Autodesk Fusion 360 part; units mm, degrees
(part 5 of 6)
sketch "Sketch13" plane through (0, 0, 0) normal (0, -1, 0) x (1, 0, 0)
  line L0 (140.1031, 86.5919) -> (126.1031, 86.5919)
  line L1 (126.1031, 86.5919) -> (126.1031, 100.5919)
  line L2 (126.1031, 100.5919) -> (140.1031, 100.5919)
  line L3 (140.1031, 100.5919) -> (140.1031, 86.5919)
  line L4 (30.8531, 93.7533) -> (30.8531, 107.7533)
  line L5 (30.8531, 107.7533) -> (44.8531, 107.7533)
  line L6 (44.8531, 107.7533) -> (44.8531, 93.7533)
  line L7 (44.8531, 93.7533) -> (30.8531, 93.7533)
  line L8 (126.1031, 67.5419) -> (126.1031, 81.5419)
  line L9 (126.1031, 81.5419) -> (140.1031, 81.5419)
  line L10 (140.1031, 81.5419) -> (140.1031, 67.5419)
  line L11 (140.1031, 67.5419) -> (126.1031, 67.5419)
  line L12 (49.9031, 98.5158) -> (49.9031, 112.5158)
  line L13 (49.9031, 112.5158) -> (63.9031, 112.5158)
  line L14 (63.9031, 112.5158) -> (63.9031, 98.5158)
  line L15 (63.9031, 98.5158) -> (49.9031, 98.5158)
  line L16 (107.0531, 96.1169) -> (107.0531, 110.1169)
  line L17 (107.0531, 110.1169) -> (121.0531, 110.1169)
  line L18 (121.0531, 110.1169) -> (121.0531, 96.1169)
  line L19 (121.0531, 96.1169) -> (107.0531, 96.1169)
  line L20 (11.8031, 93.7533) -> (11.8031, 107.7533)
  line L21 (11.8031, 107.7533) -> (25.8031, 107.7533)
  line L22 (25.8031, 107.7533) -> (25.8031, 93.7533)
  line L23 (25.8031, 93.7533) -> (11.8031, 93.7533)
  line L24 (49.9031, 41.3658) -> (49.9031, 55.3658)
  line L25 (49.9031, 55.3658) -> (63.9031, 55.3658)
  line L26 (63.9031, 55.3658) -> (63.9031, 41.3658)
  line L27 (63.9031, 41.3658) -> (49.9031, 41.3658)
  line L28 (30.8531, 74.7033) -> (30.8531, 88.7033)
  line L29 (30.8531, 88.7033) -> (44.8531, 88.7033)
  line L30 (44.8531, 88.7033) -> (44.8531, 74.7033)
  line L31 (44.8531, 74.7033) -> (30.8531, 74.7033)
  line L32 (30.8531, 55.6533) -> (30.8531, 69.6533)
  line L33 (30.8531, 69.6533) -> (44.8531, 69.6533)
  line L34 (44.8531, 69.6533) -> (44.8531, 55.6533)
  line L35 (44.8531, 55.6533) -> (30.8531, 55.6533)
  line L36 (11.8031, 17.5533) -> (11.8031, 31.5533)
  line L37 (11.8031, 31.5533) -> (25.8031, 31.5533)
  line L38 (25.8031, 31.5533) -> (25.8031, 17.5533)
  line L39 (25.8031, 17.5533) -> (11.8031, 17.5533)
  line L40 (116.8975, 10.2287) -> (104.7731, 17.2287)
  line L41 (104.7731, 17.2287) -> (106.7731, 20.6928)
  line L42 (106.7731, 20.6928) -> (104.9761, 21.7303)
  line L43 (104.9761, 21.7303) -> (103.3761, 18.959)
  line L44 (103.3761, 18.959) -> (98.3098, 21.884)
  line L45 (98.3098, 21.884) -> (104.5098, 32.6227)
  line L46 (104.5098, 32.6227) -> (109.5761, 29.6977)
  line L47 (109.5761, 29.6977) -> (107.9761, 26.9264)
  line L48 (107.9761, 26.9264) -> (109.7731, 25.8889)
  line L49 (109.7731, 25.8889) -> (111.7731, 29.353)
  line L50 (111.7731, 29.353) -> (123.8975, 22.353)
  line L51 (123.8975, 22.353) -> (121.8975, 18.8889)
  line L52 (121.8975, 18.8889) -> (123.6945, 17.8514)
  line L53 (123.6945, 17.8514) -> (125.2945, 20.6227)
  line L54 (125.2945, 20.6227) -> (130.3607, 17.6977)
  line L55 (130.3607, 17.6977) -> (124.1607, 6.959)
  line L56 (124.1607, 6.959) -> (119.0945, 9.884)
  line L57 (119.0945, 9.884) -> (120.6945, 12.6553)
  line L58 (120.6945, 12.6553) -> (118.8975, 13.6928)
  line L59 (118.8975, 13.6928) -> (116.8975, 10.2287)
  line L60 (30.8531, 36.6033) -> (30.8531, 50.6033)
  line L61 (30.8531, 50.6033) -> (44.8531, 50.6033)
  line L62 (44.8531, 50.6033) -> (44.8531, 36.6033)
  line L63 (44.8531, 36.6033) -> (30.8531, 36.6033)
  line L64 (11.8031, 36.6033) -> (11.8031, 50.6033)
  line L65 (11.8031, 50.6033) -> (25.8031, 50.6033)
  line L66 (25.8031, 50.6033) -> (25.8031, 36.6033)
  line L67 (25.8031, 36.6033) -> (11.8031, 36.6033)
  line L68 (11.8031, 55.6533) -> (11.8031, 69.6533)
  line L69 (11.8031, 69.6533) -> (25.8031, 69.6533)
  line L70 (25.8031, 69.6533) -> (25.8031, 55.6533)
  line L71 (25.8031, 55.6533) -> (11.8031, 55.6533)
  line L72 (11.8031, 74.7033) -> (11.8031, 88.7033)
  line L73 (11.8031, 88.7033) -> (25.8031, 88.7033)
  line L74 (25.8031, 88.7033) -> (25.8031, 74.7033)
  line L75 (25.8031, 74.7033) -> (11.8031, 74.7033)
  line L76 (134.7127, 21.9762) -> (122.5884, 28.9762)
  line L77 (122.5884, 28.9762) -> (129.5884, 41.1005)
  line L78 (129.5884, 41.1005) -> (141.7127, 34.1005)
  line L79 (141.7127, 34.1005) -> (134.7127, 21.9762)
  line L80 (141.6977, -4.0941) -> (129.5734, 2.9059)
  line L81 (129.5734, 2.9059) -> (136.5734, 15.0302)
  line L82 (136.5734, 15.0302) -> (148.6977, 8.0302)
  line L83 (148.6977, 8.0302) -> (141.6977, -4.0941)
  line L84 (30.8531, 17.5533) -> (30.8531, 31.5533)
  line L85 (30.8531, 31.5533) -> (44.8531, 31.5533)
  line L86 (44.8531, 31.5533) -> (44.8531, 17.5533)
  line L87 (44.8531, 17.5533) -> (30.8531, 17.5533)
  line L88 (49.9031, 22.3158) -> (49.9031, 36.3158)
  line L89 (49.9031, 36.3158) -> (63.9031, 36.3158)
  line L90 (63.9031, 36.3158) -> (63.9031, 22.3158)
  line L91 (63.9031, 22.3158) -> (49.9031, 22.3158)
  line L92 (68.9531, 100.8794) -> (68.9531, 114.8794)
  line L93 (68.9531, 114.8794) -> (82.9531, 114.8794)
  line L94 (82.9531, 114.8794) -> (82.9531, 100.8794)
  line L95 (82.9531, 100.8794) -> (68.9531, 100.8794)
  line L96 (68.9531, 81.8294) -> (68.9531, 95.8294)
  line L97 (68.9531, 95.8294) -> (82.9531, 95.8294)
  line L98 (82.9531, 95.8294) -> (82.9531, 81.8294)
  line L99 (82.9531, 81.8294) -> (68.9531, 81.8294)
  line L100 (68.9531, 62.7794) -> (68.9531, 76.7794)
  line L101 (68.9531, 76.7794) -> (82.9531, 76.7794)
  line L102 (82.9531, 76.7794) -> (82.9531, 62.7794)
  line L103 (82.9531, 62.7794) -> (68.9531, 62.7794)
  line L104 (68.9531, 43.7294) -> (68.9531, 57.7294)
  line L105 (68.9531, 57.7294) -> (82.9531, 57.7294)
  line L106 (82.9531, 57.7294) -> (82.9531, 43.7294)
  line L107 (82.9531, 43.7294) -> (68.9531, 43.7294)
  line L108 (76.5731, 22.3158) -> (76.5731, 36.3158)
  line L109 (76.5731, 36.3158) -> (90.5731, 36.3158)
  line L110 (90.5731, 36.3158) -> (90.5731, 22.3158)
  line L111 (90.5731, 22.3158) -> (76.5731, 22.3158)
  line L112 (49.9031, 60.4158) -> (49.9031, 74.4158)
  line L113 (49.9031, 74.4158) -> (63.9031, 74.4158)
  line L114 (63.9031, 74.4158) -> (63.9031, 60.4158)
  line L115 (63.9031, 60.4158) -> (49.9031, 60.4158)
  line L116 (49.9031, 79.4658) -> (49.9031, 93.4658)
  line L117 (49.9031, 93.4658) -> (63.9031, 93.4658)
  line L118 (63.9031, 93.4658) -> (63.9031, 79.4658)
  line L119 (63.9031, 79.4658) -> (49.9031, 79.4658)
  line L120 (126.1031, 48.4919) -> (126.1031, 62.4919)
  line L121 (126.1031, 62.4919) -> (140.1031, 62.4919)
  line L122 (140.1031, 62.4919) -> (140.1031, 48.4919)
  line L123 (140.1031, 48.4919) -> (126.1031, 48.4919)
  line L124 (88.0031, 60.4158) -> (88.0031, 74.4158)
  line L125 (88.0031, 74.4158) -> (102.0031, 74.4158)
  line L126 (102.0031, 74.4158) -> (102.0031, 60.4158)
  line L127 (102.0031, 60.4158) -> (88.0031, 60.4158)
  line L128 (107.0531, 91.0669) -> (121.0531, 91.0669)
  line L129 (121.0531, 91.0669) -> (121.0531, 77.0669)
  line L130 (121.0531, 77.0669) -> (107.0531, 77.0669)
  line L131 (107.0531, 77.0669) -> (107.0531, 91.0669)
  line L132 (88.0031, 79.4658) -> (88.0031, 93.4658)
  line L133 (88.0031, 93.4658) -> (102.0031, 93.4658)
  line L134 (102.0031, 93.4658) -> (102.0031, 79.4658)
  line L135 (102.0031, 79.4658) -> (88.0031, 79.4658)
  line L136 (107.0531, 58.0169) -> (107.0531, 72.0169)
  line L137 (107.0531, 72.0169) -> (121.0531, 72.0169)
  line L138 (121.0531, 72.0169) -> (121.0531, 58.0169)
  line L139 (121.0531, 58.0169) -> (107.0531, 58.0169)
  line L140 (107.0531, 38.9669) -> (107.0531, 52.9669)
  line L141 (107.0531, 52.9669) -> (121.0531, 52.9669)
  line L142 (121.0531, 52.9669) -> (121.0531, 38.9669)
  line L143 (121.0531, 38.9669) -> (107.0531, 38.9669)
  line L144 (88.0031, 41.3658) -> (88.0031, 55.3658)
  line L145 (88.0031, 55.3658) -> (102.0031, 55.3658)
  line L146 (102.0031, 55.3658) -> (102.0031, 41.3658)
  line L147 (102.0031, 41.3658) -> (88.0031, 41.3658)
  circle A0 centre (71.0494, 18.8031) radius 1.1
  line L148 (102.0031, 112.5158) -> (102.0031, 98.5158)
  line L149 (102.0031, 98.5158) -> (88.0031, 98.5158)
  line L150 (88.0031, 98.5158) -> (88.0031, 112.5158)
  line L151 (88.0031, 112.5158) -> (102.0031, 112.5158)
  circle A1 centre (18.8031, 34.0783) radius 1.1
  circle A2 centre (28.3281, 91.2283) radius 1.1
  circle A3 centre (95.25, 34.2547) radius 1.1
  circle A4 centre (115.7464, 33.7256) radius 1.1
  circle A5 centre (146.7556, 76.7997) radius 1.1
  circle A6 centre (157.6917, 44.4147) radius 1.1
  circle A7 centre (146.7556, 37.8883) radius 1.1
  line L152 (151.2227, 12.4159) -> (139.0984, 19.4159)
  line L153 (139.0984, 19.4159) -> (146.0984, 31.5402)
  line L154 (146.0984, 31.5402) -> (158.2227, 24.5402)
  line L155 (158.2227, 24.5402) -> (151.2227, 12.4159)
  circle A8 centre (123.5781, 102.5878) radius 1.1
  circle A9 centre (66.4281, 78.105) radius 1.1
  circle A10 centre (130.9158, 10.2658) radius 1.1
  arc A11 (142.7339, 99.2011) -> (138.7122, 103.2228) centre (138.7122, 99.2011) ccw
  line L156 (138.7122, 103.2228) -> (132.5162, 103.2228)
  arc A12 (131.5417, 103.3426) -> (132.5162, 103.2228) centre (132.5162, 107.2444) ccw
  line L157 (131.5417, 103.3426) -> (126.6957, 104.553)
  arc A13 (123.6486, 108.4548) -> (126.6957, 104.553) centre (127.6703, 108.4548) ccw
  line L158 (123.6486, 108.4548) -> (123.6486, 112.6772)
  line L159 (123.6486, 112.6772) -> (84.9842, 117.4397)
  line L160 (84.9842, 117.4397) -> (66.9572, 117.4397)
  line L161 (66.9572, 117.4397) -> (9.2428, 110.3136)
  line L162 (9.2428, 110.3136) -> (9.2428, 14.9931)
  line L163 (9.2428, 14.9931) -> (103.8578, 14.9931)
  line L164 (103.8578, 14.9931) -> (142.6281, -7.5847)
  line L165 (142.6281, -7.5847) -> (161.7839, 25.5411)
  arc A14 (150.7772, 34.2581) -> (152.8134, 30.7285) centre (154.8544, 34.2581) ccw
  line L166 (150.7772, 34.2581) -> (150.7772, 36.2632)
  arc A15 (154.8573, 40.3375) -> (150.7772, 36.2632) centre (154.8544, 36.2603) ccw
  line L167 (154.8573, 40.3375) -> (157.6917, 40.3375)
  arc A16 (157.6917, 40.3375) -> (157.6917, 48.4919) centre (157.6917, 44.4147) ccw
  line L168 (157.6917, 48.4919) -> (146.8111, 48.4919)
  arc A17 (142.7339, 52.5692) -> (146.8111, 48.4919) centre (146.8111, 52.5692) ccw
  line L169 (142.7339, 52.5692) -> (142.7339, 68.7564)
  arc A18 (146.7556, 72.7781) -> (142.7339, 68.7564) centre (146.7556, 68.7564) ccw
  arc A19 (146.7556, 72.7781) -> (146.7556, 80.8214) centre (146.7556, 76.7997) ccw
  arc A20 (142.7339, 84.843) -> (146.7556, 80.8214) centre (146.7556, 84.843) ccw
  line L170 (142.7339, 84.843) -> (142.7339, 99.2011)
  circle A21 centre (239.7, 32.1911) radius 17.4978
  circle A22 centre (239.7, 32.1911) radius 22.2956
  circle A23 centre (243.8628, 51.6644) radius 1.5169
  circle A24 centre (254.8342, 19.2794) radius 1.5169
  circle A25 centre (243.8628, 12.7531) radius 1.5169
  line L171 (239.7, 32.1911) -> (239.7, -10)
  line L172 (239.7, 32.1911) -> (243.8628, 12.7531)
  line L173 (239.7, 32.1911) -> (254.8342, 19.2794)
  line L174 (239.7, 32.1911) -> (243.8628, 51.6644)
  circle A26 centre (141.6031, 57.8929) radius 24.599
  circle A27 centre (141.6031, 57.8929) radius 17.5
  circle A28 centre (146.7556, 76.7997) radius 1.1
  circle A29 centre (157.6917, 44.4147) radius 1.1
  circle A30 centre (146.7556, 37.8883) radius 1.1
  line L175 (141.6031, 57.8929) -> (141.6031, 33.2939)
  line L176 (146.7556, 76.7997) -> (141.6031, 57.8929)
  line L177 (146.7556, 37.8883) -> (141.6031, 57.8929)
  line L178 (141.6031, 57.8929) -> (124.1031, 57.8929)
  line L179 (141.6031, 57.8929) -> (161.7839, 57.8929)
  line L180 (161.7839, 103.1522) -> (161.7839, 25.5411)
  line L181 (161.7839, 71.9587) -> (161.7839, 43.8272)
  line L182 (161.7839, 43.8272) -> (161.7839, 25.5411)
  line L183 (123.0531, 54.9669) -> (123.0531, 36.9669)
  line L184 (123.0531, 74.0169) -> (123.0531, 56.0169)
  line L185 (124.1031, 57.8929) -> (124.1031, 75.1805)
  line L186 (147.8246, 34.0937) -> (132.8531, 42.7375)
  line L187 (128.8563, 43.8326) -> (144.4448, 34.8326)
  line L188 (105.0531, 74.0169) -> (123.0531, 74.0169)
  line L189 (105.0531, 54.9669) -> (123.0531, 54.9669)
  line L190 (123.0531, 56.0169) -> (105.0531, 56.0169)
  line L191 (142.1031, 84.5919) -> (124.1031, 84.5919)
  line L192 (130.661, 82.4919) -> (167, 82.4919)
  point P0 (257.1978, 32.1911)
  point P1 (261.9956, 32.1911)
  point P2 (245.3797, 51.6644)
  point P3 (256.3511, 19.2794)
  point P4 (245.3797, 12.7531)
  point P5 (124.1031, 57.8929)
  dimension "d564" = 34.9956
  dimension "d565" = 44.5911
  dimension "d566" = 12.088
  dimension "d567" = 49.531
  dimension "d568" = 167.934
  dimension "d570" = 35
  dimension "d582" = 1.05
  dimension "d583" = 1.05
  dimension "d584" = 1.05
  dimension "d585" = 2.1
  constraint coincident A21.centre A22.centre
  constraint vertical L171
  constraint coincident A25.centre L172.end
  constraint coincident A24.centre L173.end
  constraint coincident A23.centre L174.end
  constraint concentric A26 A27
  constraint coincident A26.centre A27.centre
  constraint coincident A26 L175.end
  constraint parallel L169 L175
  constraint coincident A5.centre A19.centre
  constraint coincident A7.centre A30.centre
  constraint perpendicular L120 L178
  constraint perpendicular L175 L179
  constraint coincident L179.end L180
  constraint coincident L180 L181.start
  constraint coincident A26 L181.start
  constraint coincident L180 L181.end
  constraint coincident A26 L181.end
  constraint coincident A27 P5
  constraint coincident L178 P5
  constraint coincident P5 L178.end
  constraint coincident A26 L185.end
  constraint tangent A27 L185
  constraint perpendicular L178 L185
  constraint parallel L186 L187
  constraint coincident A27 L186.end
  constraint coincident A26 L186.start
  constraint tangent A27 L186
  constraint perpendicular L10 L192
  constraint tangent A26 L192
  measures "d564" diameter of A21
  measures "d565" diameter of A22
  measures "d566" angle of L171 L172
  measures "d567" angle of L171 L173
  measures "d568" angle of L171 L174
  measures "d570" diameter of A27
  measures "d582" distance of L189 L190
  measures "d583" distance of L184 L185
  measures "d584" distance of L186 L187
  measures "d585" distance of L191 L192
extrude "Extrude10" add sketch "Sketch13" against normal blind 1.2 from surface at 9.7 separate body contours L8 L11 A26 A27 L185 | L8 L9 L10 L11 A26 A27 | L9 L10 A19 A20 A26 A27 | A19 A20 A26 A27 L179 L180 L181 | A16 L168 A26 A27 L179 L180 L181 | A27 L175 L186 | L166 A15 L167 A16 L168 A26 A27 L175 L186 | L166 A15 L167 A16 A26 makes body 47
fillet "Fillet1" radius 0.5 2 edges at (124.1031, -9.1, 57.8929) (132.8531, -9.1, 42.7375) on bodies 47
sketch "Sketch14" plane through (0, 0, 0) normal (0, -1, 0) x (1, 0, 0)
  line L0 (140.1031, 86.5919) -> (126.1031, 86.5919)
  line L1 (126.1031, 86.5919) -> (126.1031, 100.5919)
  line L2 (126.1031, 100.5919) -> (140.1031, 100.5919)
  line L3 (140.1031, 100.5919) -> (140.1031, 86.5919)
  line L4 (30.8531, 93.7533) -> (30.8531, 107.7533)
  line L5 (30.8531, 107.7533) -> (44.8531, 107.7533)
  line L6 (44.8531, 107.7533) -> (44.8531, 93.7533)
  line L7 (44.8531, 93.7533) -> (30.8531, 93.7533)
  line L8 (126.1031, 67.5419) -> (126.1031, 81.5419)
  line L9 (126.1031, 81.5419) -> (140.1031, 81.5419)
  line L10 (140.1031, 81.5419) -> (140.1031, 67.5419)
  line L11 (140.1031, 67.5419) -> (126.1031, 67.5419)
  line L12 (49.9031, 98.5158) -> (49.9031, 112.5158)
  line L13 (49.9031, 112.5158) -> (63.9031, 112.5158)
  line L14 (63.9031, 112.5158) -> (63.9031, 98.5158)
  line L15 (63.9031, 98.5158) -> (49.9031, 98.5158)
  line L16 (107.0531, 96.1169) -> (107.0531, 110.1169)
  line L17 (107.0531, 110.1169) -> (121.0531, 110.1169)
  line L18 (121.0531, 110.1169) -> (121.0531, 96.1169)
  line L19 (121.0531, 96.1169) -> (107.0531, 96.1169)
  line L20 (11.8031, 93.7533) -> (11.8031, 107.7533)
  line L21 (11.8031, 107.7533) -> (25.8031, 107.7533)
  line L22 (25.8031, 107.7533) -> (25.8031, 93.7533)
  line L23 (25.8031, 93.7533) -> (11.8031, 93.7533)
  line L24 (49.9031, 41.3658) -> (49.9031, 55.3658)
  line L25 (49.9031, 55.3658) -> (63.9031, 55.3658)
  line L26 (63.9031, 55.3658) -> (63.9031, 41.3658)
  line L27 (63.9031, 41.3658) -> (49.9031, 41.3658)
  line L28 (30.8531, 74.7033) -> (30.8531, 88.7033)
  line L29 (30.8531, 88.7033) -> (44.8531, 88.7033)
  line L30 (44.8531, 88.7033) -> (44.8531, 74.7033)
  line L31 (44.8531, 74.7033) -> (30.8531, 74.7033)
  line L32 (30.8531, 55.6533) -> (30.8531, 69.6533)
  line L33 (30.8531, 69.6533) -> (44.8531, 69.6533)
  line L34 (44.8531, 69.6533) -> (44.8531, 55.6533)
  line L35 (44.8531, 55.6533) -> (30.8531, 55.6533)
  line L36 (11.8031, 17.5533) -> (11.8031, 31.5533)
  line L37 (11.8031, 31.5533) -> (25.8031, 31.5533)
  line L38 (25.8031, 31.5533) -> (25.8031, 17.5533)
  line L39 (25.8031, 17.5533) -> (11.8031, 17.5533)
  line L40 (116.8975, 10.2287) -> (104.7731, 17.2287)
  line L41 (104.7731, 17.2287) -> (106.7731, 20.6928)
  line L42 (106.7731, 20.6928) -> (104.9761, 21.7303)
  line L43 (104.9761, 21.7303) -> (103.3761, 18.959)
  line L44 (103.3761, 18.959) -> (98.3098, 21.884)
  line L45 (98.3098, 21.884) -> (104.5098, 32.6227)
  line L46 (104.5098, 32.6227) -> (109.5761, 29.6977)
  line L47 (109.5761, 29.6977) -> (107.9761, 26.9264)
  line L48 (107.9761, 26.9264) -> (109.7731, 25.8889)
  line L49 (109.7731, 25.8889) -> (111.7731, 29.353)
  line L50 (111.7731, 29.353) -> (123.8975, 22.353)
  line L51 (123.8975, 22.353) -> (121.8975, 18.8889)
  line L52 (121.8975, 18.8889) -> (123.6945, 17.8514)
  line L53 (123.6945, 17.8514) -> (125.2945, 20.6227)
  line L54 (125.2945, 20.6227) -> (130.3607, 17.6977)
  line L55 (130.3607, 17.6977) -> (124.1607, 6.959)
  line L56 (124.1607, 6.959) -> (119.0945, 9.884)
  line L57 (119.0945, 9.884) -> (120.6945, 12.6553)
  line L58 (120.6945, 12.6553) -> (118.8975, 13.6928)
  line L59 (118.8975, 13.6928) -> (116.8975, 10.2287)
  line L60 (30.8531, 36.6033) -> (30.8531, 50.6033)
  line L61 (30.8531, 50.6033) -> (44.8531, 50.6033)
  line L62 (44.8531, 50.6033) -> (44.8531, 36.6033)
  line L63 (44.8531, 36.6033) -> (30.8531, 36.6033)
  line L64 (11.8031, 36.6033) -> (11.8031, 50.6033)
  line L65 (11.8031, 50.6033) -> (25.8031, 50.6033)
  line L66 (25.8031, 50.6033) -> (25.8031, 36.6033)
  line L67 (25.8031, 36.6033) -> (11.8031, 36.6033)
  line L68 (11.8031, 55.6533) -> (11.8031, 69.6533)
  line L69 (11.8031, 69.6533) -> (25.8031, 69.6533)
  line L70 (25.8031, 69.6533) -> (25.8031, 55.6533)
  line L71 (25.8031, 55.6533) -> (11.8031, 55.6533)
  line L72 (11.8031, 74.7033) -> (11.8031, 88.7033)
  line L73 (11.8031, 88.7033) -> (25.8031, 88.7033)
  line L74 (25.8031, 88.7033) -> (25.8031, 74.7033)
  line L75 (25.8031, 74.7033) -> (11.8031, 74.7033)
  line L76 (134.7127, 21.9762) -> (122.5884, 28.9762)
  line L77 (122.5884, 28.9762) -> (129.5884, 41.1005)
  line L78 (129.5884, 41.1005) -> (141.7127, 34.1005)
  line L79 (141.7127, 34.1005) -> (134.7127, 21.9762)
  line L80 (141.6977, -4.0941) -> (129.5734, 2.9059)
  line L81 (129.5734, 2.9059) -> (136.5734, 15.0302)
  line L82 (136.5734, 15.0302) -> (148.6977, 8.0302)
  line L83 (148.6977, 8.0302) -> (141.6977, -4.0941)
  line L84 (30.8531, 17.5533) -> (30.8531, 31.5533)
  line L85 (30.8531, 31.5533) -> (44.8531, 31.5533)
  line L86 (44.8531, 31.5533) -> (44.8531, 17.5533)
  line L87 (44.8531, 17.5533) -> (30.8531, 17.5533)
  line L88 (49.9031, 22.3158) -> (49.9031, 36.3158)
  line L89 (49.9031, 36.3158) -> (63.9031, 36.3158)
  line L90 (63.9031, 36.3158) -> (63.9031, 22.3158)
  line L91 (63.9031, 22.3158) -> (49.9031, 22.3158)
  line L92 (68.9531, 100.8794) -> (68.9531, 114.8794)
  line L93 (68.9531, 114.8794) -> (82.9531, 114.8794)
  line L94 (82.9531, 114.8794) -> (82.9531, 100.8794)
  line L95 (82.9531, 100.8794) -> (68.9531, 100.8794)
  line L96 (68.9531, 81.8294) -> (68.9531, 95.8294)
  line L97 (68.9531, 95.8294) -> (82.9531, 95.8294)
  line L98 (82.9531, 95.8294) -> (82.9531, 81.8294)
  line L99 (82.9531, 81.8294) -> (68.9531, 81.8294)
  line L100 (68.9531, 62.7794) -> (68.9531, 76.7794)
  line L101 (68.9531, 76.7794) -> (82.9531, 76.7794)
  line L102 (82.9531, 76.7794) -> (82.9531, 62.7794)
  line L103 (82.9531, 62.7794) -> (68.9531, 62.7794)
  line L104 (68.9531, 43.7294) -> (68.9531, 57.7294)
  line L105 (68.9531, 57.7294) -> (82.9531, 57.7294)
  line L106 (82.9531, 57.7294) -> (82.9531, 43.7294)
  line L107 (82.9531, 43.7294) -> (68.9531, 43.7294)
  line L108 (76.5731, 22.3158) -> (76.5731, 36.3158)
  line L109 (76.5731, 36.3158) -> (90.5731, 36.3158)
  line L110 (90.5731, 36.3158) -> (90.5731, 22.3158)
  line L111 (90.5731, 22.3158) -> (76.5731, 22.3158)
  line L112 (49.9031, 60.4158) -> (49.9031, 74.4158)
  line L113 (49.9031, 74.4158) -> (63.9031, 74.4158)
  line L114 (63.9031, 74.4158) -> (63.9031, 60.4158)
  line L115 (63.9031, 60.4158) -> (49.9031, 60.4158)
  line L116 (49.9031, 79.4658) -> (49.9031, 93.4658)
  line L117 (49.9031, 93.4658) -> (63.9031, 93.4658)
  line L118 (63.9031, 93.4658) -> (63.9031, 79.4658)
  line L119 (63.9031, 79.4658) -> (49.9031, 79.4658)
  line L120 (126.1031, 48.4919) -> (126.1031, 62.4919)
  line L121 (126.1031, 62.4919) -> (140.1031, 62.4919)
  line L122 (140.1031, 62.4919) -> (140.1031, 48.4919)
  line L123 (140.1031, 48.4919) -> (126.1031, 48.4919)
  line L124 (88.0031, 60.4158) -> (88.0031, 74.4158)
  line L125 (88.0031, 74.4158) -> (102.0031, 74.4158)
  line L126 (102.0031, 74.4158) -> (102.0031, 60.4158)
  line L127 (102.0031, 60.4158) -> (88.0031, 60.4158)
  line L128 (107.0531, 91.0669) -> (121.0531, 91.0669)
  line L129 (121.0531, 91.0669) -> (121.0531, 77.0669)
  line L130 (121.0531, 77.0669) -> (107.0531, 77.0669)
  line L131 (107.0531, 77.0669) -> (107.0531, 91.0669)
  line L132 (88.0031, 79.4658) -> (88.0031, 93.4658)
  line L133 (88.0031, 93.4658) -> (102.0031, 93.4658)
  line L134 (102.0031, 93.4658) -> (102.0031, 79.4658)
  line L135 (102.0031, 79.4658) -> (88.0031, 79.4658)
  line L136 (107.0531, 58.0169) -> (107.0531, 72.0169)
  line L137 (107.0531, 72.0169) -> (121.0531, 72.0169)
  line L138 (121.0531, 72.0169) -> (121.0531, 58.0169)
  line L139 (121.0531, 58.0169) -> (107.0531, 58.0169)
  line L140 (107.0531, 38.9669) -> (107.0531, 52.9669)
  line L141 (107.0531, 52.9669) -> (121.0531, 52.9669)
  line L142 (121.0531, 52.9669) -> (121.0531, 38.9669)
  line L143 (121.0531, 38.9669) -> (107.0531, 38.9669)
  line L144 (88.0031, 41.3658) -> (88.0031, 55.3658)
  line L145 (88.0031, 55.3658) -> (102.0031, 55.3658)
  line L146 (102.0031, 55.3658) -> (102.0031, 41.3658)
  line L147 (102.0031, 41.3658) -> (88.0031, 41.3658)
  circle A0 centre (71.0494, 18.8031) radius 1.1
  line L148 (102.0031, 112.5158) -> (102.0031, 98.5158)
  line L149 (102.0031, 98.5158) -> (88.0031, 98.5158)
  line L150 (88.0031, 98.5158) -> (88.0031, 112.5158)
  line L151 (88.0031, 112.5158) -> (102.0031, 112.5158)
  circle A1 centre (18.8031, 34.0783) radius 1.1
  circle A2 centre (28.3281, 91.2283) radius 1.1
  circle A3 centre (95.25, 34.2547) radius 1.1
  circle A4 centre (115.7464, 33.7256) radius 1.1
  circle A5 centre (146.7556, 76.7997) radius 1.1
  circle A6 centre (157.6917, 44.4147) radius 1.1
  circle A7 centre (146.7556, 37.8883) radius 1.1
  line L152 (151.2227, 12.4159) -> (139.0984, 19.4159)
  line L153 (139.0984, 19.4159) -> (146.0984, 31.5402)
  line L154 (146.0984, 31.5402) -> (158.2227, 24.5402)
  line L155 (158.2227, 24.5402) -> (151.2227, 12.4159)
  circle A8 centre (123.5781, 102.5878) radius 1.1
  circle A9 centre (66.4281, 78.105) radius 1.1
  circle A10 centre (130.9158, 10.2658) radius 1.1
  arc A11 (142.7339, 99.2011) -> (138.7122, 103.2228) centre (138.7122, 99.2011) ccw
  line L156 (138.7122, 103.2228) -> (132.5162, 103.2228)
  arc A12 (131.5417, 103.3426) -> (132.5162, 103.2228) centre (132.5162, 107.2444) ccw
  line L157 (131.5417, 103.3426) -> (126.6957, 104.553)
  arc A13 (123.6486, 108.4548) -> (126.6957, 104.553) centre (127.6703, 108.4548) ccw
  line L158 (123.6486, 108.4548) -> (123.6486, 112.6772)
  line L159 (123.6486, 112.6772) -> (84.9842, 117.4397)
  line L160 (84.9842, 117.4397) -> (66.9572, 117.4397)
  line L161 (66.9572, 117.4397) -> (9.2428, 110.3136)
  line L162 (9.2428, 110.3136) -> (9.2428, 14.9931)
  line L163 (9.2428, 14.9931) -> (103.8578, 14.9931)
  line L164 (103.8578, 14.9931) -> (142.6281, -7.5847)
  line L165 (142.6281, -7.5847) -> (161.7839, 25.5411)
  line L166 (161.7839, 25.5411) -> (152.8134, 30.7285)
  arc A14 (150.7772, 34.2581) -> (152.8134, 30.7285) centre (154.8544, 34.2581) ccw
  line L167 (150.7772, 34.2581) -> (150.7772, 36.2632)
  arc A15 (154.8573, 40.3375) -> (150.7772, 36.2632) centre (154.8544, 36.2603) ccw
  line L168 (154.8573, 40.3375) -> (157.6917, 40.3375)
  arc A16 (157.6917, 40.3375) -> (157.6917, 48.4919) centre (157.6917, 44.4147) ccw
  line L169 (157.6917, 48.4919) -> (146.8111, 48.4919)
  arc A17 (142.7339, 52.5692) -> (146.8111, 48.4919) centre (146.8111, 52.5692) ccw
  line L170 (142.7339, 52.5692) -> (142.7339, 68.7564)
  arc A18 (146.7556, 72.7781) -> (142.7339, 68.7564) centre (146.7556, 68.7564) ccw
  arc A19 (146.7556, 72.7781) -> (146.7556, 80.8214) centre (146.7556, 76.7997) ccw
  arc A20 (142.7339, 84.843) -> (146.7556, 80.8214) centre (146.7556, 84.843) ccw
  line L171 (142.7339, 84.843) -> (142.7339, 99.2011)
  line L172 (146.8111, 48.4919) -> (126.1031, 48.4919)
  line L173 (126.1031, 48.4919) -> (126.1031, 72.7781)
  line L174 (126.1031, 72.7781) -> (146.7556, 72.7781)
  line L175 (126.1031, 81.5419) -> (126.1031, 67.5419)
  line L176 (140.1031, 81.5419) -> (126.1031, 81.5419)
  line L177 (140.1031, 67.5419) -> (140.1031, 81.5419)
  line L178 (126.1031, 67.5419) -> (140.1031, 67.5419)
  line L179 (126.1031, 62.4919) -> (126.1031, 48.4919)
  line L180 (140.1031, 62.4919) -> (126.1031, 62.4919)
  line L181 (140.1031, 48.4919) -> (140.1031, 62.4919)
  line L182 (126.1031, 48.4919) -> (140.1031, 48.4919)
  arc A21 (126.1031, 52.5692) -> (130.1802, 48.4919) centre (130.1803, 52.5692) ccw
  arc A22 (130.1803, 72.7781) -> (126.1031, 68.7008) centre (130.1803, 68.7008) ccw
  dimension "d588" = 4.0772
  dimension "d589" = 4.0772
  dimension "d590" = 4.0772
  constraint coincident L169.end A17.end
  constraint tangent A17 L172
  constraint perpendicular L121 L173
  constraint coincident A18.start A19.start
  constraint perpendicular L173 L174
  constraint coincident L123 A21.end
  constraint coincident L173 A21.start
  constraint tangent L172 A21
  constraint tangent L173 A21
  constraint coincident L173 L120.end
  constraint coincident L174 A22.start
  constraint coincident L173 A22.end
  constraint tangent L173 A22
  constraint tangent L174 A22
  measures "d588" radius of A17
  measures "d589" radius of A21
  measures "d590" radius of A22
extrude "Extrude1'" cut sketch "Sketch14" against normal blind 1.2 contours L10 L11 L121 L122 A17 L170 A18 L172 L173 L174 L177 L178 L180 L181 bodies 44 in component "top plate"
extrude "Extrude2'" add sketch "Sketch14" against normal blind 1.2 contours L8 L173 L174 L175 A22 | L8 L9 L10 L174 L175 L176 L177 | L120 L123 L172 L173 L179 L182 A21 bodies 44 in component "top plate"
sketch "Sketch15" plane through (0, 0, 0) normal (0, -1, 0) x (1, 0, 0)
  line L0 (130.1803, 72.7781) -> (146.7556, 72.7781)
  arc A0 (146.7556, 72.7781) -> (146.7556, 80.8214) centre (146.7556, 76.7997) ccw
  arc A1 (142.7339, 84.843) -> (146.7556, 80.8214) centre (146.7556, 84.843) ccw
  line L1 (142.7339, 84.843) -> (142.7339, 99.2011)
  arc A2 (142.7339, 99.2011) -> (138.7122, 103.2228) centre (138.7122, 99.2011) ccw
  line L2 (138.7122, 103.2228) -> (132.5162, 103.2228)
  arc A3 (131.5417, 103.3426) -> (132.5162, 103.2228) centre (132.5162, 107.2444) ccw
  line L3 (131.5417, 103.3426) -> (126.6957, 104.553)
  arc A4 (123.6486, 108.4548) -> (126.6957, 104.553) centre (127.6703, 108.4548) ccw
  line L4 (123.6486, 108.4548) -> (123.6486, 112.6772)
  line L5 (123.6486, 112.6772) -> (84.9842, 117.4397)
  line L6 (84.9842, 117.4397) -> (66.9572, 117.4397)
  line L7 (66.9572, 117.4397) -> (9.2428, 110.3136)
  line L8 (9.2428, 110.3136) -> (9.2428, 14.9931)
  line L9 (9.2428, 14.9931) -> (103.8578, 14.9931)
  line L10 (103.8578, 14.9931) -> (142.6281, -7.5847)
  line L11 (142.6281, -7.5847) -> (161.7839, 25.5411)
  line L12 (161.7839, 25.5411) -> (152.8134, 30.7285)
  arc A5 (150.7772, 34.2581) -> (152.8134, 30.7285) centre (154.8544, 34.2581) ccw
  line L13 (150.7772, 34.2581) -> (150.7772, 36.2632)
  arc A6 (154.8573, 40.3375) -> (150.7772, 36.2632) centre (154.8544, 36.2603) ccw
  line L14 (154.8573, 40.3375) -> (157.6917, 40.3375)
  arc A7 (157.6917, 40.3375) -> (157.6917, 48.4919) centre (157.6917, 44.4147) ccw
  line L15 (157.6917, 48.4919) -> (130.1802, 48.4919)
  arc A8 (126.1031, 52.5692) -> (130.1802, 48.4919) centre (130.1803, 52.5692) ccw
  line L16 (126.1031, 52.5692) -> (126.1031, 68.7008)
  arc A9 (130.1803, 72.7781) -> (126.1031, 68.7008) centre (130.1803, 68.7008) ccw
  circle A10 centre (130.9158, 10.2658) radius 1.1
  circle A11 centre (66.4281, 78.105) radius 1.1
  circle A12 centre (123.5781, 102.5878) radius 1.1
  line L17 (151.2227, 12.4159) -> (139.0984, 19.4159)
  line L18 (139.0984, 19.4159) -> (146.0984, 31.5402)
  line L19 (146.0984, 31.5402) -> (158.2227, 24.5402)
  line L20 (158.2227, 24.5402) -> (151.2227, 12.4159)
  circle A13 centre (146.7556, 37.8883) radius 1.1
  circle A14 centre (157.6917, 44.4147) radius 1.1
  circle A15 centre (146.7556, 76.7997) radius 1.1
  circle A16 centre (115.7464, 33.7256) radius 1.1
  circle A17 centre (95.25, 34.2547) radius 1.1
  circle A18 centre (28.3281, 91.2283) radius 1.1
  circle A19 centre (18.8031, 34.0783) radius 1.1
  line L21 (102.0031, 112.5158) -> (102.0031, 98.5158)
  line L22 (102.0031, 98.5158) -> (88.0031, 98.5158)
  line L23 (88.0031, 98.5158) -> (88.0031, 112.5158)
  line L24 (88.0031, 112.5158) -> (102.0031, 112.5158)
  circle A20 centre (71.0494, 18.8031) radius 1.1
  line L25 (88.0031, 41.3658) -> (88.0031, 55.3658)
  line L26 (88.0031, 55.3658) -> (102.0031, 55.3658)
  line L27 (102.0031, 55.3658) -> (102.0031, 41.3658)
  line L28 (102.0031, 41.3658) -> (88.0031, 41.3658)
  line L29 (107.0531, 38.9669) -> (107.0531, 52.9669)
  line L30 (107.0531, 52.9669) -> (121.0531, 52.9669)
  line L31 (121.0531, 52.9669) -> (121.0531, 38.9669)
  line L32 (121.0531, 38.9669) -> (107.0531, 38.9669)
  line L33 (107.0531, 58.0169) -> (107.0531, 72.0169)
  line L34 (107.0531, 72.0169) -> (121.0531, 72.0169)
  line L35 (121.0531, 72.0169) -> (121.0531, 58.0169)
  line L36 (121.0531, 58.0169) -> (107.0531, 58.0169)
  line L37 (88.0031, 79.4658) -> (88.0031, 93.4658)
  line L38 (88.0031, 93.4658) -> (102.0031, 93.4658)
  line L39 (102.0031, 93.4658) -> (102.0031, 79.4658)
  line L40 (102.0031, 79.4658) -> (88.0031, 79.4658)
  line L41 (107.0531, 91.0669) -> (121.0531, 91.0669)
  line L42 (121.0531, 91.0669) -> (121.0531, 77.0669)
  line L43 (121.0531, 77.0669) -> (107.0531, 77.0669)
  line L44 (107.0531, 77.0669) -> (107.0531, 91.0669)
  line L45 (88.0031, 60.4158) -> (88.0031, 74.4158)
  line L46 (88.0031, 74.4158) -> (102.0031, 74.4158)
  line L47 (102.0031, 74.4158) -> (102.0031, 60.4158)
  line L48 (102.0031, 60.4158) -> (88.0031, 60.4158)
  line L49 (49.9031, 79.4658) -> (49.9031, 93.4658)
  line L50 (49.9031, 93.4658) -> (63.9031, 93.4658)
  line L51 (63.9031, 93.4658) -> (63.9031, 79.4658)
  line L52 (63.9031, 79.4658) -> (49.9031, 79.4658)
  line L53 (49.9031, 60.4158) -> (49.9031, 74.4158)
  line L54 (49.9031, 74.4158) -> (63.9031, 74.4158)
  line L55 (63.9031, 74.4158) -> (63.9031, 60.4158)
  line L56 (63.9031, 60.4158) -> (49.9031, 60.4158)
  line L57 (76.5731, 22.3158) -> (76.5731, 36.3158)
  line L58 (76.5731, 36.3158) -> (90.5731, 36.3158)
  line L59 (90.5731, 36.3158) -> (90.5731, 22.3158)
  line L60 (90.5731, 22.3158) -> (76.5731, 22.3158)
  line L61 (68.9531, 43.7294) -> (68.9531, 57.7294)
  line L62 (68.9531, 57.7294) -> (82.9531, 57.7294)
  line L63 (82.9531, 57.7294) -> (82.9531, 43.7294)
  line L64 (82.9531, 43.7294) -> (68.9531, 43.7294)
  line L65 (68.9531, 62.7794) -> (68.9531, 76.7794)
  line L66 (68.9531, 76.7794) -> (82.9531, 76.7794)
  line L67 (82.9531, 76.7794) -> (82.9531, 62.7794)
  line L68 (82.9531, 62.7794) -> (68.9531, 62.7794)
  line L69 (68.9531, 81.8294) -> (68.9531, 95.8294)
  line L70 (68.9531, 95.8294) -> (82.9531, 95.8294)
  line L71 (82.9531, 95.8294) -> (82.9531, 81.8294)
  line L72 (82.9531, 81.8294) -> (68.9531, 81.8294)
  line L73 (68.9531, 100.8794) -> (68.9531, 114.8794)
  line L74 (68.9531, 114.8794) -> (82.9531, 114.8794)
  line L75 (82.9531, 114.8794) -> (82.9531, 100.8794)
  line L76 (82.9531, 100.8794) -> (68.9531, 100.8794)
  line L77 (49.9031, 22.3158) -> (49.9031, 36.3158)
  line L78 (49.9031, 36.3158) -> (63.9031, 36.3158)
  line L79 (63.9031, 36.3158) -> (63.9031, 22.3158)
  line L80 (63.9031, 22.3158) -> (49.9031, 22.3158)
  line L81 (30.8531, 17.5533) -> (30.8531, 31.5533)
  line L82 (30.8531, 31.5533) -> (44.8531, 31.5533)
  line L83 (44.8531, 31.5533) -> (44.8531, 17.5533)
  line L84 (44.8531, 17.5533) -> (30.8531, 17.5533)
  line L85 (141.6977, -4.0941) -> (129.5734, 2.9059)
  line L86 (129.5734, 2.9059) -> (136.5734, 15.0302)
  line L87 (136.5734, 15.0302) -> (148.6977, 8.0302)
  line L88 (148.6977, 8.0302) -> (141.6977, -4.0941)
  line L89 (134.7127, 21.9762) -> (122.5884, 28.9762)
  line L90 (122.5884, 28.9762) -> (129.5884, 41.1005)
  line L91 (129.5884, 41.1005) -> (141.7127, 34.1005)
  line L92 (141.7127, 34.1005) -> (134.7127, 21.9762)
  line L93 (11.8031, 74.7033) -> (11.8031, 88.7033)
  line L94 (11.8031, 88.7033) -> (25.8031, 88.7033)
  line L95 (25.8031, 88.7033) -> (25.8031, 74.7033)
  line L96 (25.8031, 74.7033) -> (11.8031, 74.7033)
  line L97 (11.8031, 55.6533) -> (11.8031, 69.6533)
  line L98 (11.8031, 69.6533) -> (25.8031, 69.6533)
  line L99 (25.8031, 69.6533) -> (25.8031, 55.6533)
  line L100 (25.8031, 55.6533) -> (11.8031, 55.6533)
  line L101 (11.8031, 36.6033) -> (11.8031, 50.6033)
  line L102 (11.8031, 50.6033) -> (25.8031, 50.6033)
  line L103 (25.8031, 50.6033) -> (25.8031, 36.6033)
  line L104 (25.8031, 36.6033) -> (11.8031, 36.6033)
  line L105 (30.8531, 36.6033) -> (30.8531, 50.6033)
  line L106 (30.8531, 50.6033) -> (44.8531, 50.6033)
  line L107 (44.8531, 50.6033) -> (44.8531, 36.6033)
  line L108 (44.8531, 36.6033) -> (30.8531, 36.6033)
  line L109 (116.8975, 10.2287) -> (104.7731, 17.2287)
  line L110 (104.7731, 17.2287) -> (106.7731, 20.6928)
  line L111 (106.7731, 20.6928) -> (104.9761, 21.7303)
  line L112 (104.9761, 21.7303) -> (103.3761, 18.959)
  line L113 (103.3761, 18.959) -> (98.3098, 21.884)
  line L114 (98.3098, 21.884) -> (104.5098, 32.6227)
  line L115 (104.5098, 32.6227) -> (109.5761, 29.6977)
  line L116 (109.5761, 29.6977) -> (107.9761, 26.9264)
  line L117 (107.9761, 26.9264) -> (109.7731, 25.8889)
  line L118 (109.7731, 25.8889) -> (111.7731, 29.353)
  line L119 (111.7731, 29.353) -> (123.8975, 22.353)
  line L120 (123.8975, 22.353) -> (121.8975, 18.8889)
  line L121 (121.8975, 18.8889) -> (123.6945, 17.8514)
  line L122 (123.6945, 17.8514) -> (125.2945, 20.6227)
  line L123 (125.2945, 20.6227) -> (130.3607, 17.6977)
  line L124 (130.3607, 17.6977) -> (124.1607, 6.959)
  line L125 (124.1607, 6.959) -> (119.0945, 9.884)
  line L126 (119.0945, 9.884) -> (120.6945, 12.6553)
  line L127 (120.6945, 12.6553) -> (118.8975, 13.6928)
  line L128 (118.8975, 13.6928) -> (116.8975, 10.2287)
  line L129 (11.8031, 17.5533) -> (11.8031, 31.5533)
  line L130 (11.8031, 31.5533) -> (25.8031, 31.5533)
  line L131 (25.8031, 31.5533) -> (25.8031, 17.5533)
  line L132 (25.8031, 17.5533) -> (11.8031, 17.5533)
  line L133 (30.8531, 55.6533) -> (30.8531, 69.6533)
  line L134 (30.8531, 69.6533) -> (44.8531, 69.6533)
  line L135 (44.8531, 69.6533) -> (44.8531, 55.6533)
  line L136 (44.8531, 55.6533) -> (30.8531, 55.6533)
  line L137 (30.8531, 74.7033) -> (30.8531, 88.7033)
  line L138 (30.8531, 88.7033) -> (44.8531, 88.7033)
  line L139 (44.8531, 88.7033) -> (44.8531, 74.7033)
  line L140 (44.8531, 74.7033) -> (30.8531, 74.7033)
  line L141 (49.9031, 41.3658) -> (49.9031, 55.3658)
  line L142 (49.9031, 55.3658) -> (63.9031, 55.3658)
  line L143 (63.9031, 55.3658) -> (63.9031, 41.3658)
  line L144 (63.9031, 41.3658) -> (49.9031, 41.3658)
  line L145 (11.8031, 93.7533) -> (11.8031, 107.7533)
  line L146 (11.8031, 107.7533) -> (25.8031, 107.7533)
  line L147 (25.8031, 107.7533) -> (25.8031, 93.7533)
  line L148 (25.8031, 93.7533) -> (11.8031, 93.7533)
  line L149 (107.0531, 96.1169) -> (107.0531, 110.1169)
  line L150 (107.0531, 110.1169) -> (121.0531, 110.1169)
  line L151 (121.0531, 110.1169) -> (121.0531, 96.1169)
  line L152 (121.0531, 96.1169) -> (107.0531, 96.1169)
  line L153 (49.9031, 98.5158) -> (49.9031, 112.5158)
  line L154 (49.9031, 112.5158) -> (63.9031, 112.5158)
  line L155 (63.9031, 112.5158) -> (63.9031, 98.5158)
  line L156 (63.9031, 98.5158) -> (49.9031, 98.5158)
  line L157 (30.8531, 93.7533) -> (30.8531, 107.7533)
  line L158 (30.8531, 107.7533) -> (44.8531, 107.7533)
  line L159 (44.8531, 107.7533) -> (44.8531, 93.7533)
  line L160 (44.8531, 93.7533) -> (30.8531, 93.7533)
  line L161 (140.1031, 86.5919) -> (126.1031, 86.5919)
  line L162 (126.1031, 86.5919) -> (126.1031, 100.5919)
  line L163 (126.1031, 100.5919) -> (140.1031, 100.5919)
  line L164 (140.1031, 100.5919) -> (140.1031, 86.5919)
  line L165 (76.5731, 36.3158) -> (76.5731, 22.3158)
  line L166 (90.5731, 36.3158) -> (76.5731, 36.3158)
  line L167 (90.5731, 22.3158) -> (90.5731, 36.3158)
  line L168 (76.5731, 22.3158) -> (90.5731, 22.3158)
  line L169 (68.9531, 43.7294) -> (82.9531, 43.7294)
  line L170 (63.9031, 22.3158) -> (63.9031, 36.3158)
  line L171 (68.9531, 38.6794) -> (82.9531, 38.6794)
  line L172 (82.9531, 38.6794) -> (82.9531, 24.6794)
  line L173 (82.9531, 24.6794) -> (68.9531, 24.6794)
  line L174 (68.9531, 24.6794) -> (68.9531, 38.6794)
  point P0 (63.9031, 41.3658)
  dimension "d595" = 5.05
  dimension "d596" = 14
  dimension "d597" = 5.05
  dimension "d598" = 5.05
  dimension "d599" = 14
  dimension "d600" = 14
  constraint horizontal L171
  constraint vertical L172
  constraint horizontal L173
  constraint vertical L174
  measures "d595" distance of L78.end P0
  measures "d596" distance of L79.end L78.end
  measures "d597" distance of L170 L174
  measures "d598" distance of L169 L171
  measures "d599" distance of L172.end L173.end
  measures "d600" distance of L171.start L173.end
extrude "Extrude3'" add sketch "Sketch15" against normal up to surface (1.2 mm away) contours L57 L58 L59 L60 L165 L166 L167 L168 L172 L173 | L57 L58 L165 L166 L172 L173 bodies 44 in component "top plate"
extrude "Extrude4'" cut sketch "Sketch15" against normal up to surface (1.2 mm away) contours L57 L58 L165 L166 L171 L172 L173 L174 | L57 L58 L165 L166 L172 L173 bodies 44 in component "top plate"
sketch "Sketch16" plane through (0, 0, 0) normal (0, -1, 0) x (1, 0, 0)
  line L0 (98.3098, 21.884) -> (104.5098, 32.6227)
  line L1 (104.5098, 32.6227) -> (109.5761, 29.6977)
  line L2 (109.5761, 29.6977) -> (107.9761, 26.9264)
  line L3 (107.9761, 26.9264) -> (109.7731, 25.8889)
  line L4 (109.7731, 25.8889) -> (111.7731, 29.353)
  line L5 (111.7731, 29.353) -> (123.8975, 22.353)
  line L6 (123.8975, 22.353) -> (121.8975, 18.8889)
  line L7 (123.6945, 17.8514) -> (125.2945, 20.6227)
  line L8 (121.8975, 18.8889) -> (123.6945, 17.8514)
  line L9 (125.2945, 20.6227) -> (130.3607, 17.6977)
  line L10 (130.3607, 17.6977) -> (124.1607, 6.959)
  line L11 (124.1607, 6.959) -> (119.0945, 9.884)
  line L12 (119.0945, 9.884) -> (120.6945, 12.6553)
  line L13 (120.6945, 12.6553) -> (118.8975, 13.6928)
  line L14 (118.8975, 13.6928) -> (116.8975, 10.2287)
  line L15 (116.8975, 10.2287) -> (104.7731, 17.2287)
  line L16 (104.7731, 17.2287) -> (106.7731, 20.6928)
  line L17 (106.7731, 20.6928) -> (104.9761, 21.7303)
  line L18 (104.9761, 21.7303) -> (103.3761, 18.959)
  line L19 (103.3761, 18.959) -> (98.3098, 21.884)
  line L20 (134.7127, 21.9762) -> (122.5884, 28.9762)
  line L21 (151.2227, 12.4159) -> (139.0984, 19.4159)
  line L22 (129.5734, 2.9059) -> (136.5734, 15.0302)
  line L23 (49.9031, 36.3158) -> (63.9031, 36.3158)
  line L24 (63.9031, 41.3658) -> (49.9031, 41.3658)
  line L25 (132.1757, 17.5692) -> (120.0513, 24.5692)
  line L26 (120.0513, 24.5692) -> (113.0513, 12.4449)
  line L27 (113.0513, 12.4449) -> (125.1757, 5.4449)
  line L28 (125.1757, 5.4449) -> (132.1757, 17.5692)
  line L29 (115.6537, 27.1082) -> (103.5293, 34.1082)
  line L30 (103.5293, 34.1082) -> (96.5293, 21.9839)
  line L31 (96.5293, 21.9839) -> (108.6537, 14.9839)
  line L32 (108.6537, 14.9839) -> (115.6537, 27.1082)
  line L33 (141.7127, 34.1005) -> (134.7127, 21.9762)
  line L34 (136.5734, 15.0302) -> (148.6977, 8.0302)
  point P0 (109.7731, 25.8889)
  point P1 (134.7127, 21.9762)
  point P2 (139.0984, 19.4159)
  point P3 (136.5734, 15.0302)
  dimension "d605" = 5.0783
  dimension "d606" = 5.0606
  dimension "d607" = 5.05
  dimension "d608" = 14
  dimension "d609" = 14
  dimension "d610" = 14
  dimension "d612" = 14
  dimension "d613" = 14
  dimension "d614" = 5.078
  dimension "d615" = 5.078
  constraint parallel L5 L27
  constraint parallel L29 L31
  constraint parallel L20 L25
  constraint parallel L20 L29
  constraint parallel L28 L33
  constraint parallel L32 L33
  constraint parallel L30 L33
  constraint parallel L26 L33
  constraint collinear L25 L34
  constraint collinear L25 L29
  measures "d605" distance of P1 P2
  measures "d606" distance of P2 P3
  measures "d607" distance of L23 L24
  measures "d608" distance of P1 L20.end
  measures "d609" distance of L26.end L27.end
  measures "d610" distance of L30.end L31.end
  measures "d612" distance of L29.start L31.end
  measures "d613" distance of L25.start L27.end
  measures "d614" distance of L22 L28
  measures "d615" distance of L26 L32
extrude "Extrude5'" add sketch "Sketch15" sketch "Sketch16" along normal up to surface contours L109 L110 L111 L112 L113 L114 L115 L116 L117 L118 L119 L120 L121 L122 L123 L124 L125 L126 L127 L128 of sketch 2 contours L0 L1 L2 L3 L4 L15 L16 L17 L18 L19 L29 L32 | L4 L5 L6 L15 L25 L26 L29 L32 end surface through (0, 1.2, 0) normal (0, 1, 0) offset 0 bodies 44 in component "top plate"
extrude "Extrude6'" cut sketch "Sketch16" against normal up to surface (1.2 mm away) contours L0 L1 L2 L3 L4 L15 L16 L17 L18 L19 L29 L30 L31 L32 | L0 L1 L2 L3 L4 L15 L16 L17 L18 L19 L29 L32 | L6 L7 L8 L9 L10 L11 L12 L13 L14 L15 L25 L26 | L6 L7 L8 L9 L10 L11 L12 L13 L14 L15 L25 L26 L27 L28 bodies 44 in component "top plate"
sketch "Sketch17" plane through (0, -9.7, 0) normal (0, -1, 0) x (1, 0, 0)
  circle A0 centre (146.7556, 76.7997) radius 1.1
  circle A1 centre (157.6917, 44.4147) radius 1.1
  circle A2 centre (146.7556, 37.8883) radius 1.1
  arc A3 (138.3203, 40.7036) -> (137.9765, 39.7794) centre (138.2265, 40.2125) ccw
  line L0 (137.9765, 39.7794) -> (147.8246, 34.0937)
  arc A4 (147.8246, 34.0937) -> (161.7839, 43.8272) centre (141.6031, 57.8929) ccw
  line L1 (161.7839, 43.8272) -> (161.7839, 71.9587)
  arc A5 (161.7839, 71.9587) -> (124.1031, 75.1805) centre (141.6031, 57.8929) ccw
  line L2 (124.1031, 75.1805) -> (124.1031, 63.809)
  arc A6 (124.1031, 63.809) -> (125.0753, 63.6447) centre (124.6031, 63.809) ccw
  arc A7 (138.3203, 40.7036) -> (125.0753, 63.6447) centre (141.6031, 57.8929) ccw
  line L3 (158.6031, 53.7396) -> (158.6031, 62.0462)
  line L4 (124.6031, 62.0462) -> (124.6031, 54)
  arc A8 (158.6031, 53.7396) -> (158.6031, 62.0462) centre (141.6031, 57.8929) ccw
  line L5 (141.6031, 57.8929) -> (141.6031, 75.3929)
  line L6 (141.6031, 57.8929) -> (132.2003, 72.6523)
  line L7 (141.6031, 57.8929) -> (126.8437, 67.2957)
  line L8 (141.6031, 57.8929) -> (153.9774, 45.5186)
  circle A9 centre (153.6239, 45.8721) radius 0.5
  circle A10 centre (154.3224, 46.0929) radius 0.15
  circle A11 centre (153.4031, 45.1736) radius 0.15
  line L9 (153.2703, 45.5186) -> (153.6188, 45.1701)
  line L10 (153.9774, 46.2257) -> (154.3259, 45.8772)
  circle A12 centre (132.8357, 72.8647) radius 0.15
  line L11 (132.8907, 72.4992) -> (132.6259, 72.9149)
  circle A13 centre (132.469, 72.2306) radius 0.5
  line L12 (132.0473, 71.9619) -> (131.7825, 72.3776)
  circle A14 centre (131.7393, 72.1663) radius 0.15
  circle A15 centre (126.6312, 66.6603) radius 0.15
  line L13 (126.9968, 66.6053) -> (126.5811, 66.8701)
  circle A16 centre (127.2654, 67.027) radius 0.5
  line L14 (127.5341, 67.4487) -> (127.1184, 67.7135)
  circle A17 centre (127.3297, 67.7567) radius 0.15
  dimension "d620" = 34
  dimension "d621" = 17
  dimension "d622" = 8.3066
  dimension "d623" = 32.5
  dimension "d624" = 25
  dimension "d625" = 135
  dimension "d626" = 1
  dimension "d627" = 0.3
  dimension "d628" = 0.3
  dimension "d629" = 1
  dimension "d630" = 0.4929
  dimension "d631" = 0.4929
  dimension "d633" = 167.5
  dimension "d635" = 25
  constraint coincident A7 L3.start
  constraint coincident A7 L3.end
  constraint parallel L2 L3
  constraint coincident A7 L4.start
  constraint parallel L3 L4
  constraint coincident A4.centre A5.centre
  constraint coincident A7 L5.end
  constraint vertical L5
  constraint coincident A7 L6.end
  constraint coincident A7 L7.end
  constraint coincident A7 L8.end
  constraint coincident L8 A9.centre
  constraint tangent A7 A9
  constraint tangent A7 A11
  constraint coincident A9 L9.start
  constraint coincident A7 L9.end
  constraint tangent A9 L9
  constraint coincident A9 L10.start
  constraint coincident A7 L10.end
  constraint parallel L9 L10
  constraint tangent A7 A10
  constraint tangent A10 L10
  constraint tangent A11 L9
  measures "d620" distance of L3 L4
  measures "d621" distance of A4.centre L3
  measures "d622" distance of L3.start L3.end
  measures "d623" angle of L5 L6
  measures "d624" angle of L6 L7
  measures "d625" angle of L5 L8
  measures "d626" diameter of A9
  measures "d627" diameter of A10
  measures "d628" diameter of A11
  measures "d629" distance of L9 L10
  measures "d630" distance of L9.start L9.end
  measures "d631" distance of L10.start L10.end
extrude "Extrude11" add sketch "Sketch17" against normal up to surface (1.2 mm away) contours A7 L3 A8 bodies 47